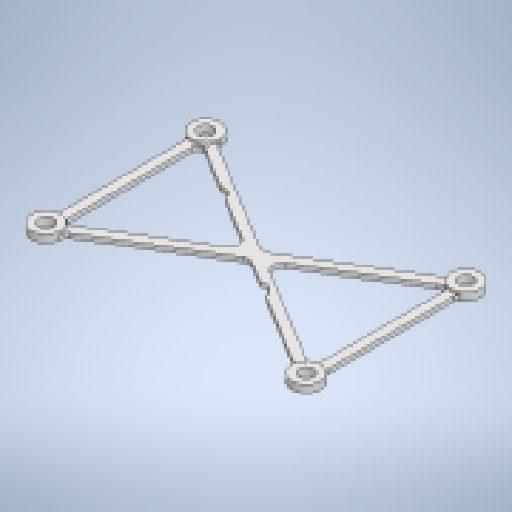
# Autodesk Inventor part: pcb_podstawka
Saved by Autodesk Inventor 2023 (Build 270158000, 158)
## iProperties
Created: 2025-03-16
Part Number: pcb_podstawka
Material: Ogólny
Document SubType Name: Modeling
Designer: kamil
Density: 1 g/cm^3
Appearance: Domyślna
Author: kamil
Autodesk Inventor part; units mm, degrees
ref_plane "YZ Plane" through (0, 0, 0) normal (1, 0, 0) x (0, 1, 0)
ref_plane "XZ Plane" through (0, 0, 0) normal (0, 1, 0) x (-1, 0, 0)
ref_plane "XY Plane" through (0, 0, 0) normal (0, 0, 1) x (1, 0, 0)
sketch "Szkic1" plane through (0, 0, 0) normal (0, 1, 0) x (-1, 0, 0)
  circle A0 centre (0, 0) radius 1.6
  circle A1 centre (0, -34.35) radius 1.6
  circle A2 centre (-56, 0) radius 1.6
  circle A3 centre (-56, -34.35) radius 1.6
  circle A4 centre (0, 0) radius 3.1
  circle A5 centre (-56, 0) radius 3.1
  circle A6 centre (0, -34.35) radius 3.1
  circle A7 centre (-56, -34.35) radius 3.1
  line L0 (0, 0) -> (0, -34.35)
  line L1 (0, -34.35) -> (-56, -34.35)
  line L2 (-56, -34.35) -> (-56, 0)
  line L3 (-56, 0) -> (0, 0)
  line L4 (1.2, -35.55) -> (1.2, 1.2)
  line L5 (1.2, 1.2) -> (-57.2, 1.2)
  line L6 (-57.2, 1.2) -> (-57.2, -35.55)
  line L7 (-57.2, -35.55) -> (1.2, -35.55)
  line L8 (-1.2, -33.15) -> (-1.2, -1.2)
  line L9 (-1.2, -1.2) -> (-54.8, -1.2)
  line L10 (-54.8, -1.2) -> (-54.8, -33.15)
  line L11 (-54.8, -33.15) -> (-1.2, -33.15)
  point P0 (1.2, -2.8583)
  point P1 (-2.8583, 1.2)
  point P2 (-53.1417, 1.2)
  point P3 (-57.2, -2.8583)
  point P4 (-57.2, -31.4917)
  point P5 (-53.1417, -35.55)
  point P6 (-2.8583, -35.55)
  point P7 (1.2, -31.4917)
  point P8 (-1.2, -2.8583)
  point P9 (-1.2, -31.4917)
  point P10 (-2.8583, -33.15)
  point P11 (-53.1417, -33.15)
  point P12 (-54.8, -31.4917)
  point P13 (-54.8, -2.8583)
  point P14 (-53.1417, -1.2)
  point P15 (-2.8583, -1.2)
  dimension "d0" = 56
  dimension "d1" = 34.35
  dimension "d2" = 3.2
  dimension "d3" = 3.2
  dimension "d4" = 3.2
  dimension "d5" = 3.2
  dimension "d6" = 1.5
  dimension "d7" = 1.5
  dimension "d8" = 1.5
  dimension "d9" = 1.5
  dimension "d10" = 1.2
  dimension "d11" = 1.2
  constraints: 24 end point, 9 perpendicular, 8 centre point, 5 coincident, 2 horizontal alignment, 2 vertical alignment, 1 vertical, 6 other
  measures "d0" distance of point (0, 0) point (-56, 0)
  measures "d1" distance of point (0, -34.35) point (0, 0)
  measures "d2" diameter of A0
  measures "d3" diameter of A1
  measures "d4" diameter of A2
  measures "d5" diameter of A3
  measures "d6" radial gap between concentric circles of A0 A4
  measures "d7" radial gap between concentric circles of A2 A5
  measures "d8" radial gap between concentric circles of A1 A6
  measures "d9" radial gap between concentric circles of A3 A7
  measures "d10" distance between parallel lines of L0 L4
  measures "d11" distance between parallel lines of L0 L8
extrude "Wyciągnięcie proste2" add sketch "Szkic1" along normal blind 1 contours A0 L4 | A0 L4 L5 A4 | L4 A0 L0 L3 L5 | A0 L5 L4 | L4 A4 L0 A0 | L5 A0 | L0 A4 L8 L9 L3 A0 | A0 L3 L0 | A0 L3 A4 L5 | L4 A1 L0 A6 | A6 L7 A1 L4 | A4 L9 L8 | L0 A1 L1 A6 L11 L8 | L4 A1 L7 L1 L0 | A1 L4 | L5 A2 L6 A5 | A5 L3 A2 L5 | A5 L9 L10 L2 A2 L3 | L8 L11 A6 | L0 L1 A1 | A6 L1 A1 L7 | L4 L7 A1 | L6 A2 L2 A5 | L5 A2 | A2 L3 L2 L6 L5 | A5 L10 L9 | A2 L2 L3 | L7 A3 L1 A7 | A7 L6 A3 L7 | L7 A1 | A2 L6 | A7 L2 A3 L6 | A2 L6 L5 | L11 L10 A7 | A7 L1 A3 L2 L10 L11 | L7 A3 L6 L2 L1 | A3 L7 | L6 A3 | L1 L2 A3 | L7 L6 A3
sketch "Szkic2" plane through (0, 1, 0) normal (0, 1, 0) x (1, 0, 0)
  circle A0 centre (0, 0) radius 3.1 projected
  circle A1 centre (0, 34.35) radius 3.1 projected
  circle A2 centre (56, 0) radius 3.1 projected
  circle A3 centre (56, 34.35) radius 3.1 projected
hole "Otwór1" at (0, 1, 0) at (0, 1, -34.35) at (56, 1, -34.35) at (56, 1, 0) direction (0, -1, 0) diameter 3.2 depth 14 tip angle 118
sketch "Szkic3" plane through (0, 0, 0) normal (0, -1, 0) x (1, 0, 0)
  circle A0 centre (56, 0) radius 1.6 projected
  circle A1 centre (56, -34.35) radius 1.6 projected
  circle A2 centre (0, 0) radius 1.6 projected
  circle A3 centre (0, -34.35) radius 1.6 projected
  circle A4 centre (56, 0) radius 1.6 projected
  circle A5 centre (0, -34.35) radius 1.6 projected
  line L0 (56, 0) -> (0, -34.35)
  line L1 (56, -34.35) -> (0, 0)
  line L2 (55.4771, 0.8524) -> (-0.5229, -33.4976)
  line L3 (56.5229, -0.8524) -> (0.5229, -35.2024)
  line L4 (56.5229, -33.4976) -> (0.5229, 0.8524)
  line L5 (55.4771, -35.2024) -> (-0.5229, -0.8524)
  point P0 (29.9125, -17.175)
  point P1 (55.4582, -1.5055)
  point P2 (54.4125, 0.1994)
  point P3 (28, -16.0019)
  point P4 (1.5875, 0.1994)
  point P5 (0.5418, -1.5055)
  point P6 (26.0875, -17.175)
  point P7 (0.5418, -32.8445)
  point P8 (1.5875, -34.5494)
  point P9 (28, -18.3481)
  point P10 (54.4125, -34.5494)
  point P11 (55.4582, -32.8445)
  dimension "d23" = 1
  dimension "d24" = 1
  dimension "d25" = 1
  dimension "d26" = 1
  constraints: 12 end point, 4 parallel
  measures "d23" distance between parallel lines of L0 L2
  measures "d24" distance between parallel lines of L0 L3
  measures "d25" distance between parallel lines of L1 L4
  measures "d26" distance between parallel lines of L1 L5
extrude "Wyciągnięcie proste3" add sketch "Szkic3" against normal blind 0.4 contours A0 L0 L4 L2 | L3 L4 L0 A0 | L4 L0 L1 L2 | L2 L1 A2 L4 | L4 A1 L1 L3 | L3 L1 L0 L4 | L2 L5 A2 L1 | L1 L0 L5 L2 | L3 L5 L0 L1 | L1 A1 L5 L3 | L5 L0 A3 L2 | L3 A3 L0 L5
fillet "Zaokrąglenie1" radius 2 8 edges at (54.0216, 0.2, -2.3866) (52.9759, 0.2, -0.6818) (52.9759, 0.2, -33.6682) (54.0216, 0.2, -31.9634) (1.9784, 0.2, -31.9634) (3.0241, 0.2, -33.6682) (3.0241, 0.2, -0.6818) (1.9784, 0.2, -2.3866)
sketch "Szkic4" plane through (0, 0, 0) normal (0, -1, 0) x (1, 0, 0)
  circle A0 centre (0, 0) radius 1.6 projected
  circle A1 centre (0, -34.35) radius 1.6 projected
  circle A2 centre (56, -34.35) radius 1.6 projected
  circle A3 centre (56, 0) radius 1.6 projected
  line L0 (0, -34.35) -> (0, 0)
  line L1 (56, -34.35) -> (56, 0)
  line L2 (-1, -34.35) -> (-1, 0)
  line L3 (1, -34.35) -> (1, 0)
  line L4 (55, -34.35) -> (55, 0)
  line L5 (57, -34.35) -> (57, 0)
  point P0 (-1, -1.249)
  point P1 (-1, -33.101)
  point P2 (1, -33.101)
  point P3 (1, -1.249)
  point P4 (57, -33.101)
  point P5 (57, -1.249)
  point P6 (55, -1.249)
  point P7 (55, -33.101)
  dimension "d30" = 1
  dimension "d31" = 1
  dimension "d32" = 1
  dimension "d33" = 1
  constraints: 12 end point, 4 parallel, 2 vertical
  measures "d30" distance between parallel lines of L0 L2
  measures "d31" distance between parallel lines of L0 L3
  measures "d32" distance between parallel lines of L1 L4
  measures "d33" distance between parallel lines of L1 L5
extrude "Wyciągnięcie proste4" add sketch "Szkic4" against normal blind 0.4 contours A0 L0 A1 L2 | L3 A1 L0 A0 | A2 L1 A3 L5 | L4 A3 L1 A2
fillet "Zaokrąglenie2" radius 1 8 edges at (1, 0.2, -31.4157) (-1, 0.2, -31.4157) (-1, 0.2, -2.9343) (1, 0.2, -2.9343) (57, 0.2, -2.9343) (55, 0.2, -2.9343) (57, 0.2, -31.4157) (55, 0.2, -31.4157)
fillet "Zaokrąglenie3" radius 2 4 edges at (28, 0.2, -18.3481) (26.0875, 0.2, -17.175) (28, 0.2, -16.0019) (29.9125, 0.2, -17.175)
sketch "Szkic5" plane through (0, 0, 0) normal (0, -1, 0) x (1, 0, 0)
  arc A0 (2.9928, -3.0089) -> (2.053, -2.7165) centre (1.947, -4.7137) ccw projected
  line L0 (2.9928, -3.0089) -> (23.3081, -15.4702) projected
  arc A1 (23.3081, -18.8798) -> (23.3081, -15.4702) centre (22.2624, -17.175) ccw projected
  line L1 (23.3081, -18.8798) -> (2.9928, -31.3411) projected
  arc A2 (2.053, -31.6335) -> (2.9928, -31.3411) centre (1.947, -29.6363) ccw projected
  arc A3 (1, -30.6349) -> (2.053, -31.6335) centre (2, -30.6349) ccw projected
  line L2 (1, -30.6349) -> (1, -3.7151) projected
  arc A4 (2.053, -2.7165) -> (1, -3.7151) centre (2, -3.7151) ccw projected
  arc A5 (55, -3.7151) -> (53.947, -2.7165) centre (54, -3.7151) ccw projected
  line L3 (55, -3.7151) -> (55, -30.6349) projected
  arc A6 (53.947, -31.6335) -> (55, -30.6349) centre (54, -30.6349) ccw projected
  arc A7 (53.0072, -31.3411) -> (53.947, -31.6335) centre (54.053, -29.6363) ccw projected
  line L4 (53.0072, -31.3411) -> (32.6919, -18.8798) projected
  arc A8 (32.6919, -15.4702) -> (32.6919, -18.8798) centre (33.7376, -17.175) ccw projected
  line L5 (32.6919, -15.4702) -> (53.0072, -3.0089) projected
  arc A9 (53.947, -2.7165) -> (53.0072, -3.0089) centre (54.053, -4.7137) ccw projected
  line L6 (-1, -3.5791) -> (-1, -30.7709) projected
  arc A10 (-1.5122, -31.6438) -> (-1, -30.7709) centre (-2, -30.7709) ccw projected
  arc A11 (-1.5122, -31.6438) -> (3.0904, -34.5936) centre (0, -34.35) ccw projected
  arc A12 (4.0385, -33.046) -> (3.0904, -34.5936) centre (5.0842, -34.7508) ccw projected
  line L7 (4.0385, -33.046) -> (26.9543, -18.9896) projected
  arc A13 (29.0457, -18.9896) -> (26.9543, -18.9896) centre (28, -20.6944) ccw projected
  line L8 (29.0457, -18.9896) -> (51.9615, -33.046) projected
  arc A14 (52.9096, -34.5936) -> (51.9615, -33.046) centre (50.9158, -34.7508) ccw projected
  arc A15 (52.9096, -34.5936) -> (57.5122, -31.6438) centre (56, -34.35) ccw projected
  arc A16 (57, -30.7709) -> (57.5122, -31.6438) centre (58, -30.7709) ccw projected
  line L9 (57, -30.7709) -> (57, -3.5791) projected
  arc A17 (57.5122, -2.7062) -> (57, -3.5791) centre (58, -3.5791) ccw projected
  arc A18 (57.5122, -2.7062) -> (52.9096, 0.2436) centre (56, 0) ccw projected
  arc A19 (51.9615, -1.304) -> (52.9096, 0.2436) centre (50.9158, 0.4008) ccw projected
  line L10 (51.9615, -1.304) -> (29.0457, -15.3604) projected
  arc A20 (26.9543, -15.3604) -> (29.0457, -15.3604) centre (28, -13.6556) ccw projected
  line L11 (26.9543, -15.3604) -> (4.0385, -1.304) projected
  arc A21 (3.0904, 0.2436) -> (4.0385, -1.304) centre (5.0842, 0.4008) ccw projected
  arc A22 (3.0904, 0.2436) -> (-1.5122, -2.7062) centre (0, 0) ccw projected
  arc A23 (-1, -3.5791) -> (-1.5122, -2.7062) centre (-2, -3.5791) ccw projected
  circle A24 centre (0, -34.35) radius 1.6 projected
  circle A25 centre (0, 0) radius 1.6 projected
  circle A26 centre (56, 0) radius 1.6 projected
  circle A27 centre (56, -34.35) radius 1.6 projected
extrude "Wyciągnięcie proste5" add sketch "Szkic5" along normal blind 0.6
sketch "Szkic6" plane through (0, -0.6, 0) normal (0, -1, 0) x (1, 0, 0)
  line L0 (33.2848, -12.4625) -> (34.6345, -13.0599)
  line L1 (34.6345, -13.0599) -> (36.6765, -11.416)
  line L2 (36.6765, -11.416) -> (36.5335, -10.0469)
  line L3 (33.2848, -12.4625) -> (36.5335, -10.0469)
  line L4 (10.6612, -26.4098) -> (13.6267, -25.8869)
  line L5 (13.6267, -25.8869) -> (14.7365, -23.3796)
  line L6 (14.7365, -23.3796) -> (10.6612, -26.4098)
  point P0 (0, 0)
  constraints: 14 end point, 1 parallel
extrude "Wyciągnięcie proste6" cut sketch "Szkic6" against normal through all
